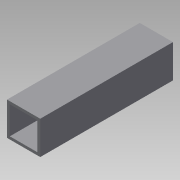
# Autodesk Inventor part: body_frame
Saved by Autodesk Inventor 2015 (Build 190159000, 159)
## iProperties
Created: 2014-06-09
Part Number: body_frame
Material: Generic
Document SubType Name: Modeling
Designer: L
Density: 1 g/cm^3
Appearance: Default
Mass: 540.773 g
Surface Area: 1738.71 cm^2
Volume: 540.773 cm^3
Author: L
Autodesk Inventor part; units mm, degrees
ref_plane "YZ Plane" through (0, 0, 0) normal (1, 0, 0) x (0, 1, 0)
ref_plane "XZ Plane" through (0, 0, 0) normal (0, 1, 0) x (-1, 0, 0)
ref_plane "XY Plane" through (0, 0, 0) normal (0, 0, 1) x (1, 0, 0)
sketch "Sketch1" plane through (0, 0, 0) normal (0, 0, 1) x (1, 0, 0)
  line L0 (-38.1, -38.1) -> (38.1, -38.1)
  line L1 (38.1, -38.1) -> (38.1, 38.1)
  line L2 (38.1, 38.1) -> (-38.1, 38.1)
  line L3 (-38.1, 38.1) -> (-38.1, -38.1)
  line L4 (-38.1, -38.1) -> (38.1, 38.1) construction
  line L5 (38.1, -38.1) -> (-38.1, 38.1) construction
  line L6 (-31.75, -31.75) -> (31.75, -31.75)
  line L7 (31.75, -31.75) -> (31.75, 31.75)
  line L8 (31.75, 31.75) -> (-31.75, 31.75)
  line L9 (-31.75, 31.75) -> (-31.75, -31.75)
  line L10 (-31.75, -31.75) -> (31.75, 31.75) construction
  line L11 (31.75, -31.75) -> (-31.75, 31.75) construction
  point P0 (0, 0)
  dimension "d0" = 76.2
  dimension "d1" = 76.2
  dimension "d2" = 63.5
  dimension "d3" = 63.5
  constraints: 24 end point, 4 midpoint, 4 parallel, 2 horizontal, 2 perpendicular
  measures "d0" distance of L2.end L1.end
  measures "d1" distance of L1.end L0.end
  measures "d2" distance of L8.end L7.end
  measures "d3" distance of L7.end L6.end
extrude "Extrusion1" add sketch "Sketch1" along normal blind 304.8
equation "\"d0\" = width"
equation "\"d1\" = width"
equation "\"d2\" = width - 2 * thickness"
equation "\"d3\" = width - 2 * thickness"
equation "\"d4\" = length"
equation "\"width\" = 76.2"
equation "\"thickness\" = 6.35"
equation "\"length\" = 304.8"
body "Solid1"
